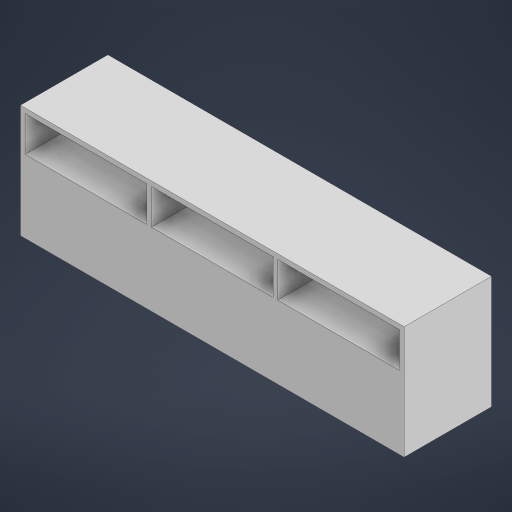
# Autodesk Inventor part: BRIMNES
Saved by Autodesk Inventor 2024.2 (Build 282272000, 272)
## iProperties
Created: 2025-08-11
Part Number: BRIMNES
Material: Generic
Document SubType Name: Modeling
Designer: Luca
Density: 1 g/cm^3
Appearance: Default
Author: Luca
Autodesk Inventor part; units mm, degrees
ref_plane "YZ Plane" through (0, 0, 0) normal (1, 0, 0) x (0, 1, 0)
ref_plane "XZ Plane" through (0, 0, 0) normal (0, 1, 0) x (-1, 0, 0)
ref_plane "XY Plane" through (0, 0, 0) normal (0, 0, 1) x (1, 0, 0)
sketch "Sketch1" plane through (0, 0, 0) normal (0, 0, 1) x (1, 0, 0)
  line L0 (-900, 530) -> (900, 530)
  line L1 (900, 530) -> (900, 0)
  line L2 (900, 0) -> (-900, 0)
  line L3 (-900, 0) -> (-900, 530)
  point P0 (0, 0)
  point P1 (0, 0)
  dimension "d0" = 1800
  dimension "d1" = 530
  constraints: 8 end point, 2 parallel, 1 coincident, 1 horizontal, 1 midpoint, 1 perpendicular
  measures "d0" distance of L1.end L2.end
  measures "d1" distance of L2.end L0.start
extrude "Extrusion1" add sketch "Sketch1" along normal blind 410
sketch "Sketch2" plane through (0, 0, 410) normal (0, 0, 1) x (1, 0, 0)
  line L0 (-877.5, 507.5) -> (-307.5, 507.5)
  line L1 (-307.5, 507.5) -> (-307.5, 342.5)
  line L2 (-307.5, 342.5) -> (-877.5, 342.5)
  line L3 (-877.5, 342.5) -> (-877.5, 507.5)
  line L4 (-285, 507.5) -> (285, 507.5)
  line L5 (285, 507.5) -> (285, 342.5)
  line L6 (285, 342.5) -> (-285, 342.5)
  line L7 (-285, 342.5) -> (-285, 507.5)
  line L8 (307.5, 507.5) -> (877.5, 507.5)
  line L9 (877.5, 507.5) -> (877.5, 342.5)
  line L10 (877.5, 342.5) -> (307.5, 342.5)
  line L11 (307.5, 342.5) -> (307.5, 507.5)
  line L12 (-900, 0) -> (900, 0) projected
  line L13 (900, 0) -> (900, 530) projected
  line L14 (900, 530) -> (-900, 530) projected
  line L15 (-900, 530) -> (-900, 0) projected
  line L16 (-900, 530) -> (-877.5, 507.5) construction
  line L17 (877.5, 507.5) -> (900, 530) construction
  point P0 (0, 0)
  point P1 (0, 342.5)
  point P2 (0, 0)
  dimension "d5" = 570
  dimension "d6" = 165
  dimension "d7" = 22.5
  dimension "d8" = 22.5
  constraints: 28 end point, 6 parallel, 4 perpendicular, 4 point on line, 3 equal length, 3 horizontal, 2 midpoint, 1 vertical alignment
  measures "d5" distance of L0.start L0.end
  measures "d6" distance between parallel lines of L0 L2
  measures "d7" distance between parallel lines of L14 L0
  measures "d8" distance between parallel lines of L7 L1
extrude "Extrusion2" cut sketch "Sketch2" against normal blind 387.5 contours L0 L1 L2 L3 | L4 L5 L6 L7 | L8 L9 L10 L11
body "Solid1"
